Autodesk Fusion 360 part; units mm, degrees
(part 3 of 6)
sketch "Sketch27" plane through (0, 0, 4) normal (0, 0, 1) x (1, 0, 0)
  arc A0 (9.3874, -0.8005) -> (9.3971, -0.6778) centre (0, 0) ccw
  spline S0 degree 3 poles (9.5677, -0.4943) (9.542, -0.4981) (9.5172, -0.5068) (9.4723, -0.5334) (9.4527, -0.5509) (9.4254, -0.587) (9.4161, -0.6039) (9.4026, -0.6398) (9.3985, -0.6587) (9.3971, -0.6778) knots 0 0 0 0 0.007813 0.007813 0.015626 0.015626 0.021388 0.021388 0.027151 0.027151 0.027151 0.027151
  spline S1 degree 5 poles (9.5677, -0.4943) (9.5692, -0.4941) (9.5738, -0.4934) (9.5816, -0.4923) (9.5926, -0.4906) (9.6069, -0.4883) (9.6229, -0.4856) (9.6389, -0.4827) (9.6549, -0.4797) (9.6709, -0.4766) (9.6869, -0.4734) (9.7029, -0.4701) (9.7189, -0.4667) (9.7349, -0.4631) (9.7509, -0.4595) (9.7669, -0.4557) (9.7829, -0.4519) (9.7989, -0.4479) (9.8149, -0.4439) (9.8309, -0.4397) (9.8469, -0.4355) (9.8629, -0.4311) (9.8788, -0.4267) (9.8948, -0.4222) (9.9108, -0.4176) (9.9268, -0.4129) (9.9428, -0.4081) (9.9587, -0.4032) (9.9747, -0.3982) (9.9906, -0.3931) (10.0066, -0.388) (10.0225, -0.3828) (10.0385, -0.3775) (10.0544, -0.3721) (10.0704, -0.3666) (10.0863, -0.3611) (10.1022, -0.3554) (10.1181, -0.3497) (10.1341, -0.3439) (10.15, -0.338) (10.1659, -0.3321) (10.1818, -0.3261) (10.1977, -0.32) (10.2136, -0.3138) (10.2294, -0.3075) (10.2453, -0.3012) (10.2612, -0.2948) (10.277, -0.2883) (10.2929, -0.2818) (10.3087, -0.2752) (10.3246, -0.2685) (10.3404, -0.2617) (10.3562, -0.2549) (10.372, -0.248) (10.3878, -0.241) (10.4036, -0.2339) (10.4194, -0.2268) (10.4352, -0.2196) (10.451, -0.2124) (10.4668, -0.205) (10.4794, -0.1991) (10.4888, -0.1946) (10.4951, -0.1917) (10.4983, -0.1902) knots 0.165068 0.165068 0.165068 0.165068 0.165068 0.165068 0.171429 0.185714 0.2 0.214286 0.228571 0.242857 0.257143 0.271429 0.285714 0.3 0.314286 0.328571 0.342857 0.357143 0.371429 0.385714 0.4 0.414286 0.428571 0.442857 0.457143 0.471429 0.485714 0.5 0.514286 0.528571 0.542857 0.557143 0.571429 0.585714 0.6 0.614286 0.628571 0.642857 0.657143 0.671429 0.685714 0.7 0.714286 0.728571 0.742857 0.757143 0.771429 0.785714 0.8 0.814286 0.828571 0.842857 0.857143 0.871429 0.885714 0.9 0.914286 0.928571 0.942857 0.957143 0.971429 0.985714 1 1 1 1 1 1
  arc A1 (10.4983, -0.1902) -> (10.4983, 0.1902) centre (0, 0) ccw
  spline S2 degree 5 poles (10.4983, 0.1902) (10.4951, 0.1917) (10.4888, 0.1946) (10.4794, 0.1991) (10.4668, 0.205) (10.451, 0.2124) (10.4352, 0.2196) (10.4194, 0.2268) (10.4036, 0.2339) (10.3878, 0.241) (10.372, 0.248) (10.3562, 0.2549) (10.3404, 0.2617) (10.3246, 0.2685) (10.3087, 0.2752) (10.2929, 0.2818) (10.277, 0.2883) (10.2612, 0.2948) (10.2453, 0.3012) (10.2294, 0.3075) (10.2136, 0.3138) (10.1977, 0.32) (10.1818, 0.3261) (10.1659, 0.3321) (10.15, 0.338) (10.1341, 0.3439) (10.1181, 0.3497) (10.1022, 0.3554) (10.0863, 0.3611) (10.0704, 0.3666) (10.0544, 0.3721) (10.0385, 0.3775) (10.0225, 0.3828) (10.0066, 0.388) (9.9906, 0.3931) (9.9747, 0.3982) (9.9587, 0.4032) (9.9428, 0.4081) (9.9268, 0.4129) (9.9108, 0.4176) (9.8948, 0.4222) (9.8788, 0.4267) (9.8629, 0.4311) (9.8469, 0.4355) (9.8309, 0.4397) (9.8149, 0.4439) (9.7989, 0.4479) (9.7829, 0.4519) (9.7669, 0.4557) (9.7509, 0.4595) (9.7349, 0.4631) (9.7189, 0.4667) (9.7029, 0.4701) (9.6869, 0.4734) (9.6709, 0.4766) (9.6549, 0.4797) (9.6389, 0.4827) (9.6229, 0.4856) (9.6069, 0.4883) (9.5926, 0.4906) (9.5816, 0.4923) (9.5738, 0.4934) (9.5692, 0.4941) (9.5677, 0.4943) knots -1 -1 -1 -1 -1 -1 -0.985714 -0.971429 -0.957143 -0.942857 -0.928571 -0.914286 -0.9 -0.885714 -0.871429 -0.857143 -0.842857 -0.828571 -0.814286 -0.8 -0.785714 -0.771429 -0.757143 -0.742857 -0.728571 -0.714286 -0.7 -0.685714 -0.671429 -0.657143 -0.642857 -0.628571 -0.614286 -0.6 -0.585714 -0.571429 -0.557143 -0.542857 -0.528571 -0.514286 -0.5 -0.485714 -0.471429 -0.457143 -0.442857 -0.428571 -0.414286 -0.4 -0.385714 -0.371429 -0.357143 -0.342857 -0.328571 -0.314286 -0.3 -0.285714 -0.271429 -0.257143 -0.242857 -0.228571 -0.214286 -0.2 -0.185714 -0.171429 -0.165068 -0.165068 -0.165068 -0.165068 -0.165068 -0.165068
  spline S3 degree 3 poles (9.3971, 0.6778) (9.399, 0.6519) (9.4059, 0.6265) (9.4291, 0.5799) (9.4451, 0.559) (9.4791, 0.5292) (9.4953, 0.5187) (9.5302, 0.5026) (9.5487, 0.4971) (9.5677, 0.4943) knots 0 0 0 0 0.007813 0.007813 0.015626 0.015626 0.021388 0.021388 0.027151 0.027151 0.027151 0.027151
  arc A2 (9.3971, 0.6778) -> (9.3874, 0.8005) centre (0, 0) ccw
  spline S4 degree 3 poles (9.5273, 1.0085) (9.5024, 1.0007) (9.4793, 0.9882) (9.4391, 0.955) (9.4225, 0.9347) (9.4012, 0.8947) (9.3947, 0.8766) (9.3869, 0.8389) (9.3858, 0.8197) (9.3874, 0.8005) knots 0 0 0 0 0.007813 0.007813 0.015626 0.015626 0.021388 0.021388 0.027151 0.027151 0.027151 0.027151
  spline S5 degree 5 poles (9.5273, 1.0085) (9.5286, 1.0089) (9.5331, 1.0103) (9.5406, 1.0127) (9.5513, 1.0161) (9.565, 1.0206) (9.5803, 1.0258) (9.5957, 1.0311) (9.6111, 1.0365) (9.6264, 1.0421) (9.6417, 1.0478) (9.657, 1.0535) (9.6722, 1.0594) (9.6875, 1.0654) (9.7027, 1.0715) (9.7179, 1.0777) (9.7331, 1.0841) (9.7483, 1.0905) (9.7635, 1.097) (9.7786, 1.1036) (9.7938, 1.1103) (9.8089, 1.1171) (9.824, 1.1239) (9.839, 1.1309) (9.8541, 1.138) (9.8691, 1.1451) (9.8842, 1.1524) (9.8992, 1.1597) (9.9142, 1.1671) (9.9291, 1.1746) (9.9441, 1.1821) (9.959, 1.1898) (9.9739, 1.1975) (9.9889, 1.2054) (10.0037, 1.2133) (10.0186, 1.2212) (10.0335, 1.2293) (10.0483, 1.2374) (10.0631, 1.2456) (10.0779, 1.2539) (10.0927, 1.2623) (10.1074, 1.2707) (10.1222, 1.2792) (10.1369, 1.2878) (10.1516, 1.2965) (10.1663, 1.3052) (10.181, 1.314) (10.1956, 1.3229) (10.2102, 1.3318) (10.2249, 1.3409) (10.2395, 1.35) (10.254, 1.3591) (10.2686, 1.3683) (10.2831, 1.3776) (10.2977, 1.387) (10.3122, 1.3964) (10.3266, 1.4059) (10.3411, 1.4155) (10.3556, 1.4252) (10.37, 1.4349) (10.3815, 1.4427) (10.3901, 1.4486) (10.3959, 1.4525) (10.3988, 1.4545) knots 0.165068 0.165068 0.165068 0.165068 0.165068 0.165068 0.171429 0.185714 0.2 0.214286 0.228571 0.242857 0.257143 0.271429 0.285714 0.3 0.314286 0.328571 0.342857 0.357143 0.371429 0.385714 0.4 0.414286 0.428571 0.442857 0.457143 0.471429 0.485714 0.5 0.514286 0.528571 0.542857 0.557143 0.571429 0.585714 0.6 0.614286 0.628571 0.642857 0.657143 0.671429 0.685714 0.7 0.714286 0.728571 0.742857 0.757143 0.771429 0.785714 0.8 0.814286 0.828571 0.842857 0.857143 0.871429 0.885714 0.9 0.914286 0.928571 0.942857 0.957143 0.971429 0.985714 1 1 1 1 1 1
  arc A3 (10.3988, 1.4545) -> (10.3393, 1.8301) centre (0, 0) ccw
  spline S6 degree 5 poles (10.3393, 1.8301) (10.3359, 1.8311) (10.3292, 1.8331) (10.3192, 1.836) (10.3058, 1.8399) (10.2891, 1.8446) (10.2724, 1.8493) (10.2557, 1.854) (10.239, 1.8585) (10.2223, 1.863) (10.2056, 1.8674) (10.1888, 1.8718) (10.1722, 1.8761) (10.1555, 1.8803) (10.1388, 1.8844) (10.1221, 1.8885) (10.1054, 1.8925) (10.0887, 1.8964) (10.072, 1.9002) (10.0554, 1.904) (10.0387, 1.9077) (10.0221, 1.9113) (10.0054, 1.9148) (9.9888, 1.9183) (9.9721, 1.9217) (9.9555, 1.925) (9.9389, 1.9282) (9.9223, 1.9314) (9.9056, 1.9345) (9.889, 1.9374) (9.8724, 1.9404) (9.8559, 1.9432) (9.8393, 1.9459) (9.8227, 1.9486) (9.8061, 1.9512) (9.7896, 1.9537) (9.773, 1.9561) (9.7565, 1.9584) (9.74, 1.9607) (9.7235, 1.9628) (9.707, 1.9649) (9.6905, 1.9668) (9.674, 1.9687) (9.6575, 1.9705) (9.6411, 1.9722) (9.6246, 1.9738) (9.6082, 1.9753) (9.5918, 1.9767) (9.5754, 1.978) (9.559, 1.9792) (9.5426, 1.9803) (9.5262, 1.9813) (9.5099, 1.9822) (9.4936, 1.983) (9.4773, 1.9836) (9.461, 1.9842) (9.4447, 1.9846) (9.4284, 1.9849) (9.4122, 1.9851) (9.3978, 1.9851) (9.3866, 1.9851) (9.3787, 1.985) (9.374, 1.985) (9.3726, 1.985) knots -1 -1 -1 -1 -1 -1 -0.985714 -0.971429 -0.957143 -0.942857 -0.928571 -0.914286 -0.9 -0.885714 -0.871429 -0.857143 -0.842857 -0.828571 -0.814286 -0.8 -0.785714 -0.771429 -0.757143 -0.742857 -0.728571 -0.714286 -0.7 -0.685714 -0.671429 -0.657143 -0.642857 -0.628571 -0.614286 -0.6 -0.585714 -0.571429 -0.557143 -0.542857 -0.528571 -0.514286 -0.5 -0.485714 -0.471429 -0.457143 -0.442857 -0.428571 -0.414286 -0.4 -0.385714 -0.371429 -0.357143 -0.342857 -0.328571 -0.314286 -0.3 -0.285714 -0.271429 -0.257143 -0.242857 -0.228571 -0.214286 -0.2 -0.185714 -0.171429 -0.165068 -0.165068 -0.165068 -0.165068 -0.165068 -0.165068
  spline S7 degree 3 poles (9.1754, 2.1395) (9.1813, 2.1142) (9.1921, 2.0902) (9.2223, 2.0478) (9.2414, 2.0297) (9.2796, 2.0056) (9.2973, 1.9977) (9.3343, 1.9873) (9.3534, 1.9847) (9.3726, 1.985) knots 0 0 0 0 0.007813 0.007813 0.015626 0.015626 0.021388 0.021388 0.027151 0.027151 0.027151 0.027151
  arc A4 (9.1754, 2.1395) -> (9.1466, 2.2592) centre (0, 0) ccw
  spline S8 degree 3 poles (9.2522, 2.4865) (9.2289, 2.4749) (9.208, 2.4589) (9.1735, 2.4199) (9.1603, 2.3971) (9.1455, 2.3544) (9.1419, 2.3354) (9.1401, 2.297) (9.142, 2.2778) (9.1466, 2.2592) knots 0 0 0 0 0.007813 0.007813 0.015626 0.015626 0.021388 0.021388 0.027151 0.027151 0.027151 0.027151
  spline S9 degree 5 poles (9.2522, 2.4865) (9.2535, 2.4871) (9.2577, 2.4892) (9.2648, 2.4927) (9.2747, 2.4977) (9.2875, 2.5043) (9.3019, 2.5118) (9.3163, 2.5195) (9.3306, 2.5273) (9.3448, 2.5351) (9.3591, 2.5431) (9.3733, 2.5513) (9.3874, 2.5595) (9.4016, 2.5678) (9.4156, 2.5762) (9.4297, 2.5847) (9.4437, 2.5933) (9.4577, 2.602) (9.4717, 2.6108) (9.4856, 2.6197) (9.4995, 2.6287) (9.5134, 2.6378) (9.5272, 2.6469) (9.541, 2.6562) (9.5548, 2.6655) (9.5685, 2.6749) (9.5822, 2.6844) (9.5959, 2.694) (9.6095, 2.7036) (9.6232, 2.7134) (9.6367, 2.7232) (9.6503, 2.7331) (9.6638, 2.7431) (9.6773, 2.7531) (9.6908, 2.7632) (9.7042, 2.7735) (9.7176, 2.7837) (9.731, 2.7941) (9.7443, 2.8045) (9.7577, 2.815) (9.7709, 2.8256) (9.7842, 2.8362) (9.7974, 2.8469) (9.8106, 2.8577) (9.8238, 2.8686) (9.8369, 2.8795) (9.8501, 2.8905) (9.8631, 2.9016) (9.8762, 2.9127) (9.8892, 2.9239) (9.9022, 2.9351) (9.9152, 2.9465) (9.9281, 2.9579) (9.941, 2.9693) (9.9539, 2.9808) (9.9667, 2.9924) (9.9796, 3.0041) (9.9924, 3.0158) (10.0051, 3.0276) (10.0178, 3.0394) (10.028, 3.0489) (10.0356, 3.0561) (10.0407, 3.0609) (10.0432, 3.0633) knots 0.165068 0.165068 0.165068 0.165068 0.165068 0.165068 0.171429 0.185714 0.2 0.214286 0.228571 0.242857 0.257143 0.271429 0.285714 0.3 0.314286 0.328571 0.342857 0.357143 0.371429 0.385714 0.4 0.414286 0.428571 0.442857 0.457143 0.471429 0.485714 0.5 0.514286 0.528571 0.542857 0.557143 0.571429 0.585714 0.6 0.614286 0.628571 0.642857 0.657143 0.671429 0.685714 0.7 0.714286 0.728571 0.742857 0.757143 0.771429 0.785714 0.8 0.814286 0.828571 0.842857 0.857143 0.871429 0.885714 0.9 0.914286 0.928571 0.942857 0.957143 0.971429 0.985714 1 1 1 1 1 1
  arc A5 (10.0432, 3.0633) -> (9.9257, 3.425) centre (0, 0) ccw
  spline S10 degree 5 poles (9.9257, 3.425) (9.9222, 3.4254) (9.9153, 3.4263) (9.9049, 3.4277) (9.8911, 3.4294) (9.8739, 3.4315) (9.8566, 3.4335) (9.8394, 3.4355) (9.8222, 3.4374) (9.805, 3.4392) (9.7878, 3.441) (9.7706, 3.4426) (9.7534, 3.4443) (9.7363, 3.4458) (9.7192, 3.4473) (9.702, 3.4487) (9.6849, 3.45) (9.6679, 3.4513) (9.6508, 3.4524) (9.6337, 3.4536) (9.6167, 3.4546) (9.5997, 3.4556) (9.5827, 3.4565) (9.5657, 3.4573) (9.5487, 3.458) (9.5318, 3.4587) (9.5149, 3.4593) (9.498, 3.4598) (9.4811, 3.4602) (9.4642, 3.4606) (9.4474, 3.4609) (9.4305, 3.4611) (9.4137, 3.4612) (9.3969, 3.4612) (9.3802, 3.4612) (9.3634, 3.4611) (9.3467, 3.4609) (9.33, 3.4606) (9.3133, 3.4602) (9.2967, 3.4597) (9.2801, 3.4592) (9.2635, 3.4586) (9.2469, 3.4578) (9.2304, 3.457) (9.2138, 3.4561) (9.1973, 3.4551) (9.1809, 3.454) (9.1644, 3.4529) (9.148, 3.4516) (9.1317, 3.4502) (9.1153, 3.4487) (9.099, 3.4471) (9.0827, 3.4455) (9.0665, 3.4437) (9.0503, 3.4418) (9.0341, 3.4398) (9.0179, 3.4377) (9.0018, 3.4354) (8.9858, 3.4331) (8.9715, 3.4308) (8.9605, 3.4291) (8.9527, 3.4278) (8.9481, 3.427) (8.9467, 3.4267) knots -1 -1 -1 -1 -1 -1 -0.985714 -0.971429 -0.957143 -0.942857 -0.928571 -0.914286 -0.9 -0.885714 -0.871429 -0.857143 -0.842857 -0.828571 -0.814286 -0.8 -0.785714 -0.771429 -0.757143 -0.742857 -0.728571 -0.714286 -0.7 -0.685714 -0.671429 -0.657143 -0.642857 -0.628571 -0.614286 -0.6 -0.585714 -0.571429 -0.557143 -0.542857 -0.528571 -0.514286 -0.5 -0.485714 -0.471429 -0.457143 -0.442857 -0.428571 -0.414286 -0.4 -0.385714 -0.371429 -0.357143 -0.342857 -0.328571 -0.314286 -0.3 -0.285714 -0.271429 -0.257143 -0.242857 -0.228571 -0.214286 -0.2 -0.185714 -0.171429 -0.165068 -0.165068 -0.165068 -0.165068 -0.165068 -0.165068
  spline S11 degree 3 poles (8.7277, 3.5485) (8.7375, 3.5244) (8.7519, 3.5024) (8.7884, 3.4652) (8.8101, 3.4504) (8.8517, 3.4325) (8.8703, 3.4275) (8.9085, 3.423) (8.9278, 3.4235) (8.9467, 3.4267) knots 0 0 0 0 0.007813 0.007813 0.015626 0.015626 0.021388 0.021388 0.027151 0.027151 0.027151 0.027151
  arc A6 (8.7277, 3.5485) -> (8.6806, 3.6622) centre (0, 0) ccw
  spline S12 degree 3 poles (8.7493, 3.9032) (8.7281, 3.8882) (8.71, 3.8691) (8.682, 3.8251) (8.6725, 3.8006) (8.6646, 3.7561) (8.664, 3.7368) (8.6683, 3.6986) (8.6731, 3.6799) (8.6806, 3.6622) knots 0 0 0 0 0.007813 0.007813 0.015626 0.015626 0.021388 0.021388 0.027151 0.027151 0.027151 0.027151
  spline S13 degree 5 poles (8.7493, 3.9032) (8.7505, 3.904) (8.7543, 3.9067) (8.7608, 3.9113) (8.7698, 3.9179) (8.7814, 3.9264) (8.7945, 3.9361) (8.8074, 3.9459) (8.8204, 3.9558) (8.8332, 3.9658) (8.846, 3.9759) (8.8588, 3.9861) (8.8715, 3.9965) (8.8841, 4.0069) (8.8967, 4.0174) (8.9093, 4.028) (8.9218, 4.0387) (8.9342, 4.0495) (8.9467, 4.0604) (8.959, 4.0713) (8.9713, 4.0824) (8.9836, 4.0935) (8.9958, 4.1047) (9.008, 4.116) (9.0202, 4.1274) (9.0323, 4.1388) (9.0443, 4.1503) (9.0563, 4.1619) (9.0683, 4.1736) (9.0802, 4.1854) (9.0921, 4.1972) (9.1039, 4.2091) (9.1157, 4.221) (9.1275, 4.2331) (9.1392, 4.2452) (9.1509, 4.2574) (9.1625, 4.2696) (9.1741, 4.282) (9.1856, 4.2943) (9.1972, 4.3068) (9.2086, 4.3193) (9.2201, 4.3319) (9.2314, 4.3445) (9.2428, 4.3573) (9.2541, 4.37) (9.2654, 4.3829) (9.2766, 4.3958) (9.2878, 4.4088) (9.299, 4.4218) (9.3101, 4.4349) (9.3211, 4.448) (9.3322, 4.4613) (9.3432, 4.4745) (9.3541, 4.4879) (9.365, 4.5013) (9.3759, 4.5147) (9.3868, 4.5282) (9.3976, 4.5418) (9.4083, 4.5554) (9.419, 4.5691) (9.4276, 4.5801) (9.434, 4.5884) (9.4382, 4.5939) (9.4404, 4.5967) knots 0.165068 0.165068 0.165068 0.165068 0.165068 0.165068 0.171429 0.185714 0.2 0.214286 0.228571 0.242857 0.257143 0.271429 0.285714 0.3 0.314286 0.328571 0.342857 0.357143 0.371429 0.385714 0.4 0.414286 0.428571 0.442857 0.457143 0.471429 0.485714 0.5 0.514286 0.528571 0.542857 0.557143 0.571429 0.585714 0.6 0.614286 0.628571 0.642857 0.657143 0.671429 0.685714 0.7 0.714286 0.728571 0.742857 0.757143 0.771429 0.785714 0.8 0.814286 0.828571 0.842857 0.857143 0.871429 0.885714 0.9 0.914286 0.928571 0.942857 0.957143 0.971429 0.985714 1 1 1 1 1 1
  arc A7 (9.4404, 4.5967) -> (9.2677, 4.9355) centre (0, 0) ccw
  spline S14 degree 5 poles (9.2677, 4.9355) (9.2642, 4.9355) (9.2572, 4.9353) (9.2468, 4.935) (9.2329, 4.9345) (9.2155, 4.9339) (9.1981, 4.9332) (9.1808, 4.9324) (9.1635, 4.9316) (9.1462, 4.9307) (9.129, 4.9297) (9.1118, 4.9287) (9.0946, 4.9276) (9.0774, 4.9265) (9.0602, 4.9252) (9.0431, 4.9239) (9.026, 4.9226) (9.0089, 4.9212) (8.9919, 4.9197) (8.9749, 4.9181) (8.9579, 4.9164) (8.9409, 4.9147) (8.924, 4.913) (8.9071, 4.9111) (8.8902, 4.9092) (8.8734, 4.9072) (8.8566, 4.9051) (8.8398, 4.903) (8.823, 4.9008) (8.8063, 4.8985) (8.7896, 4.8961) (8.773, 4.8937) (8.7564, 4.8912) (8.7398, 4.8886) (8.7232, 4.886) (8.7067, 4.8832) (8.6902, 4.8804) (8.6738, 4.8775) (8.6574, 4.8745) (8.641, 4.8715) (8.6247, 4.8683) (8.6084, 4.8651) (8.5921, 4.8618) (8.5759, 4.8584) (8.5597, 4.8549) (8.5436, 4.8514) (8.5275, 4.8477) (8.5115, 4.844) (8.4955, 4.8401) (8.4795, 4.8362) (8.4636, 4.8322) (8.4477, 4.8281) (8.4319, 4.8239) (8.4161, 4.8196) (8.4004, 4.8152) (8.3848, 4.8107) (8.3691, 4.8061) (8.3536, 4.8013) (8.3381, 4.7965) (8.3244, 4.7921) (8.3138, 4.7886) (8.3063, 4.7861) (8.3018, 4.7846) (8.3005, 4.7841) knots -1 -1 -1 -1 -1 -1 -0.985714 -0.971429 -0.957143 -0.942857 -0.928571 -0.914286 -0.9 -0.885714 -0.871429 -0.857143 -0.842857 -0.828571 -0.814286 -0.8 -0.785714 -0.771429 -0.757143 -0.742857 -0.728571 -0.714286 -0.7 -0.685714 -0.671429 -0.657143 -0.642857 -0.628571 -0.614286 -0.6 -0.585714 -0.571429 -0.557143 -0.542857 -0.528571 -0.514286 -0.5 -0.485714 -0.471429 -0.457143 -0.442857 -0.428571 -0.414286 -0.4 -0.385714 -0.371429 -0.357143 -0.342857 -0.328571 -0.314286 -0.3 -0.285714 -0.271429 -0.257143 -0.242857 -0.228571 -0.214286 -0.2 -0.185714 -0.171429 -0.165068 -0.165068 -0.165068 -0.165068 -0.165068 -0.165068
  spline S15 degree 3 poles (8.0651, 4.8702) (8.0786, 4.8479) (8.0963, 4.8284) (8.1381, 4.7974) (8.1619, 4.7861) (8.2057, 4.775) (8.2249, 4.7729) (8.2633, 4.7744) (8.2823, 4.7779) (8.3005, 4.7841) knots 0 0 0 0 0.007813 0.007813 0.015626 0.015626 0.021388 0.021388 0.027151 0.027151 0.027151 0.027151
  arc A8 (8.0651, 4.8702) -> (8.0008, 4.9751) centre (0, 0) ccw
  spline S16 degree 3 poles (8.031, 5.2238) (8.0124, 5.2057) (7.9975, 5.184) (7.9768, 5.1362) (7.9712, 5.1105) (7.9703, 5.0653) (7.9727, 5.0461) (7.9829, 5.0091) (7.9907, 4.9914) (8.0008, 4.9751) knots 0 0 0 0 0.007813 0.007813 0.015626 0.015626 0.021388 0.021388 0.027151 0.027151 0.027151 0.027151
  spline S17 degree 5 poles (8.031, 5.2238) (8.032, 5.2249) (8.0354, 5.2281) (8.041, 5.2337) (8.0489, 5.2415) (8.0591, 5.2517) (8.0705, 5.2634) (8.0817, 5.2751) (8.0929, 5.2869) (8.1041, 5.2988) (8.1151, 5.3108) (8.1261, 5.3229) (8.1371, 5.3351) (8.1479, 5.3473) (8.1587, 5.3597) (8.1695, 5.3721) (8.1801, 5.3847) (8.1908, 5.3973) (8.2013, 5.4099) (8.2118, 5.4227) (8.2223, 5.4355) (8.2326, 5.4484) (8.243, 5.4614) (8.2532, 5.4745) (8.2634, 5.4876) (8.2736, 5.5008) (8.2837, 5.5141) (8.2938, 5.5274) (8.3037, 5.5408) (8.3137, 5.5543) (8.3236, 5.5678) (8.3334, 5.5814) (8.3432, 5.5951) (8.3529, 5.6088) (8.3626, 5.6226) (8.3722, 5.6365) (8.3818, 5.6504) (8.3913, 5.6644) (8.4008, 5.6784) (8.4102, 5.6925) (8.4196, 5.7067) (8.4289, 5.7209) (8.4382, 5.7352) (8.4474, 5.7495) (8.4565, 5.7639) (8.4657, 5.7784) (8.4747, 5.7929) (8.4838, 5.8074) (8.4927, 5.822) (8.5017, 5.8367) (8.5106, 5.8514) (8.5194, 5.8662) (8.5282, 5.881) (8.5369, 5.8959) (8.5456, 5.9109) (8.5542, 5.9259) (8.5628, 5.9409) (8.5714, 5.956) (8.5799, 5.9711) (8.5883, 5.9863) (8.595, 5.9985) (8.6001, 6.0077) (8.6034, 6.0138) (8.6051, 6.0169) knots 0.165068 0.165068 0.165068 0.165068 0.165068 0.165068 0.171429 0.185714 0.2 0.214286 0.228571 0.242857 0.257143 0.271429 0.285714 0.3 0.314286 0.328571 0.342857 0.357143 0.371429 0.385714 0.4 0.414286 0.428571 0.442857 0.457143 0.471429 0.485714 0.5 0.514286 0.528571 0.542857 0.557143 0.571429 0.585714 0.6 0.614286 0.628571 0.642857 0.657143 0.671429 0.685714 0.7 0.714286 0.728571 0.742857 0.757143 0.771429 0.785714 0.8 0.814286 0.828571 0.842857 0.857143 0.871429 0.885714 0.9 0.914286 0.928571 0.942857 0.957143 0.971429 0.985714 1 1 1 1 1 1
  arc A9 (8.6051, 6.0169) -> (8.3815, 6.3246) centre (0, 0) ccw
  spline S18 degree 5 poles (8.3815, 6.3246) (8.3781, 6.3239) (8.3712, 6.3227) (8.361, 6.3207) (8.3473, 6.3181) (8.3302, 6.3147) (8.3132, 6.3113) (8.2962, 6.3079) (8.2792, 6.3044) (8.2623, 6.3008) (8.2454, 6.2971) (8.2286, 6.2934) (8.2117, 6.2897) (8.1949, 6.2858) (8.1782, 6.2819) (8.1615, 6.278) (8.1448, 6.274) (8.1282, 6.2699) (8.1116, 6.2657) (8.095, 6.2615) (8.0785, 6.2572) (8.062, 6.2529) (8.0456, 6.2485) (8.0292, 6.244) (8.0128, 6.2395) (7.9965, 6.2349) (7.9802, 6.2302) (7.964, 6.2255) (7.9478, 6.2207) (7.9316, 6.2158) (7.9155, 6.2109) (7.8994, 6.2059) (7.8834, 6.2008) (7.8674, 6.1956) (7.8515, 6.1904) (7.8356, 6.1851) (7.8198, 6.1798) (7.804, 6.1743) (7.7883, 6.1688) (7.7726, 6.1632) (7.7569, 6.1576) (7.7413, 6.1519) (7.7258, 6.146) (7.7103, 6.1402) (7.6949, 6.1342) (7.6795, 6.1282) (7.6642, 6.122) (7.6489, 6.1158) (7.6337, 6.1095) (7.6186, 6.1032) (7.6035, 6.0967) (7.5884, 6.0902) (7.5735, 6.0835) (7.5586, 6.0768) (7.5437, 6.07) (7.529, 6.0631) (7.5143, 6.0561) (7.4997, 6.049) (7.4851, 6.0418) (7.4723, 6.0353) (7.4623, 6.0302) (7.4553, 6.0265) (7.4512, 6.0244) (7.4499, 6.0237) knots -1 -1 -1 -1 -1 -1 -0.985714 -0.971429 -0.957143 -0.942857 -0.928571 -0.914286 -0.9 -0.885714 -0.871429 -0.857143 -0.842857 -0.828571 -0.814286 -0.8 -0.785714 -0.771429 -0.757143 -0.742857 -0.728571 -0.714286 -0.7 -0.685714 -0.671429 -0.657143 -0.642857 -0.628571 -0.614286 -0.6 -0.585714 -0.571429 -0.557143 -0.542857 -0.528571 -0.514286 -0.5 -0.485714 -0.471429 -0.457143 -0.442857 -0.428571 -0.414286 -0.4 -0.385714 -0.371429 -0.357143 -0.342857 -0.328571 -0.314286 -0.3 -0.285714 -0.271429 -0.257143 -0.242857 -0.228571 -0.214286 -0.2 -0.185714 -0.171429 -0.165068 -0.165068 -0.165068 -0.165068 -0.165068 -0.165068
  spline S19 degree 3 poles (7.204, 6.0719) (7.2208, 6.0519) (7.2413, 6.0355) (7.2874, 6.0114) (7.3127, 6.004) (7.3577, 5.9998) (7.377, 6.0008) (7.4147, 6.0083) (7.4329, 6.0148) (7.4499, 6.0237) knots 0 0 0 0 0.007813 0.007813 0.015626 0.015626 0.021388 0.021388 0.027151 0.027151 0.027151 0.027151
  arc A10 (7.204, 6.0719) -> (7.1241, 6.1654) centre (0, 0) ccw
  spline S20 degree 3 poles (7.1149, 6.4159) (7.0994, 6.395) (7.088, 6.3713) (7.0751, 6.3208) (7.0736, 6.2946) (7.0798, 6.2497) (7.0852, 6.2312) (7.1011, 6.1962) (7.1115, 6.18) (7.1241, 6.1654) knots 0 0 0 0 0.007813 0.007813 0.015626 0.015626 0.021388 0.021388 0.027151 0.027151 0.027151 0.027151
  spline S21 degree 5 poles (7.1149, 6.4159) (7.1158, 6.417) (7.1186, 6.4208) (7.1233, 6.4271) (7.1299, 6.4361) (7.1383, 6.4478) (7.1477, 6.4611) (7.157, 6.4744) (7.1663, 6.4878) (7.1754, 6.5013) (7.1844, 6.5149) (7.1934, 6.5286) (7.2023, 6.5423) (7.2111, 6.5561) (7.2198, 6.57) (7.2285, 6.584) (7.2371, 6.598) (7.2456, 6.6121) (7.254, 6.6263) (7.2624, 6.6405) (7.2707, 6.6549) (7.279, 6.6692) (7.2871, 6.6837) (7.2952, 6.6982) (7.3033, 6.7127) (7.3112, 6.7274) (7.3191, 6.742) (7.327, 6.7568) (7.3347, 6.7716) (7.3424, 6.7865) (7.3501, 6.8014) (7.3577, 6.8163) (7.3652, 6.8314) (7.3727, 6.8465) (7.3801, 6.8616) (7.3874, 6.8768) (7.3947, 6.892) (7.4019, 6.9073) (7.409, 6.9227) (7.4161, 6.9381) (7.4232, 6.9535) (7.4302, 6.969) (7.4371, 6.9846) (7.444, 7.0002) (7.4508, 7.0158) (7.4575, 7.0315) (7.4642, 7.0473) (7.4708, 7.0631) (7.4774, 7.0789) (7.4839, 7.0948) (7.4904, 7.1107) (7.4968, 7.1267) (7.5032, 7.1427) (7.5095, 7.1588) (7.5157, 7.1749) (7.5219, 7.1911) (7.528, 7.2073) (7.5341, 7.2235) (7.5401, 7.2398) (7.5461, 7.2561) (7.5508, 7.2692) (7.5544, 7.2791) (7.5567, 7.2857) (7.5579, 7.2889) knots 0.165068 0.165068 0.165068 0.165068 0.165068 0.165068 0.171429 0.185714 0.2 0.214286 0.228571 0.242857 0.257143 0.271429 0.285714 0.3 0.314286 0.328571 0.342857 0.357143 0.371429 0.385714 0.4 0.414286 0.428571 0.442857 0.457143 0.471429 0.485714 0.5 0.514286 0.528571 0.542857 0.557143 0.571429 0.585714 0.6 0.614286 0.628571 0.642857 0.657143 0.671429 0.685714 0.7 0.714286 0.728571 0.742857 0.757143 0.771429 0.785714 0.8 0.814286 0.828571 0.842857 0.857143 0.871429 0.885714 0.9 0.914286 0.928571 0.942857 0.957143 0.971429 0.985714 1 1 1 1 1 1
  arc A11 (7.5579, 7.2889) -> (7.2889, 7.5579) centre (0, 0) ccw
  spline S22 degree 5 poles (7.2889, 7.5579) (7.2857, 7.5567) (7.2791, 7.5544) (7.2692, 7.5508) (7.2561, 7.5461) (7.2398, 7.5401) (7.2235, 7.5341) (7.2073, 7.528) (7.1911, 7.5219) (7.1749, 7.5157) (7.1588, 7.5095) (7.1427, 7.5032) (7.1267, 7.4968) (7.1107, 7.4904) (7.0948, 7.4839) (7.0789, 7.4774) (7.0631, 7.4708) (7.0473, 7.4642) (7.0315, 7.4575) (7.0158, 7.4508) (7.0002, 7.444) (6.9846, 7.4371) (6.969, 7.4302) (6.9535, 7.4232) (6.9381, 7.4161) (6.9227, 7.409) (6.9073, 7.4019) (6.892, 7.3947) (6.8768, 7.3874) (6.8616, 7.3801) (6.8465, 7.3727) (6.8314, 7.3652) (6.8163, 7.3577) (6.8014, 7.3501) (6.7865, 7.3424) (6.7716, 7.3347) (6.7568, 7.327) (6.742, 7.3191) (6.7274, 7.3112) (6.7127, 7.3033) (6.6982, 7.2952) (6.6837, 7.2871) (6.6692, 7.279) (6.6549, 7.2707) (6.6405, 7.2624) (6.6263, 7.254) (6.6121, 7.2456) (6.598, 7.2371) (6.584, 7.2285) (6.57, 7.2198) (6.5561, 7.2111) (6.5423, 7.2023) (6.5286, 7.1934) (6.5149, 7.1844) (6.5013, 7.1754) (6.4878, 7.1663) (6.4744, 7.157) (6.4611, 7.1477) (6.4478, 7.1383) (6.4361, 7.1299) (6.4271, 7.1233) (6.4208, 7.1186) (6.417, 7.1158) (6.4159, 7.1149) knots -1 -1 -1 -1 -1 -1 -0.985714 -0.971429 -0.957143 -0.942857 -0.928571 -0.914286 -0.9 -0.885714 -0.871429 -0.857143 -0.842857 -0.828571 -0.814286 -0.8 -0.785714 -0.771429 -0.757143 -0.742857 -0.728571 -0.714286 -0.7 -0.685714 -0.671429 -0.657143 -0.642857 -0.628571 -0.614286 -0.6 -0.585714 -0.571429 -0.557143 -0.542857 -0.528571 -0.514286 -0.5 -0.485714 -0.471429 -0.457143 -0.442857 -0.428571 -0.414286 -0.4 -0.385714 -0.371429 -0.357143 -0.342857 -0.328571 -0.314286 -0.3 -0.285714 -0.271429 -0.257143 -0.242857 -0.228571 -0.214286 -0.2 -0.185714 -0.171429 -0.165068 -0.165068 -0.165068 -0.165068 -0.165068 -0.165068
  spline S23 degree 3 poles (6.1654, 7.1241) (6.1851, 7.107) (6.208, 7.094) (6.2573, 7.0774) (6.2834, 7.074) (6.3286, 7.077) (6.3474, 7.081) (6.3835, 7.0943) (6.4005, 7.1035) (6.4159, 7.1149) knots 0 0 0 0 0.007813 0.007813 0.015626 0.015626 0.021388 0.021388 0.027151 0.027151 0.027151 0.027151
  arc A12 (6.1654, 7.1241) -> (6.0719, 7.204) centre (0, 0) ccw
  spline S24 degree 3 poles (6.0237, 7.4499) (6.0116, 7.4268) (6.0041, 7.4016) (5.9992, 7.3498) (6.0018, 7.3236) (6.015, 7.2803) (6.0232, 7.2629) (6.0443, 7.2308) (6.0572, 7.2163) (6.0719, 7.204) knots 0 0 0 0 0.007813 0.007813 0.015626 0.015626 0.021388 0.021388 0.027151 0.027151 0.027151 0.027151
  spline S25 degree 5 poles (6.0237, 7.4499) (6.0244, 7.4512) (6.0265, 7.4553) (6.0302, 7.4623) (6.0353, 7.4723) (6.0418, 7.4851) (6.049, 7.4997) (6.0561, 7.5143) (6.0631, 7.529) (6.07, 7.5437) (6.0768, 7.5586) (6.0835, 7.5735) (6.0902, 7.5884) (6.0967, 7.6035) (6.1032, 7.6186) (6.1095, 7.6337) (6.1158, 7.6489) (6.122, 7.6642) (6.1282, 7.6795) (6.1342, 7.6949) (6.1402, 7.7103) (6.146, 7.7258) (6.1519, 7.7413) (6.1576, 7.7569) (6.1632, 7.7726) (6.1688, 7.7883) (6.1743, 7.804) (6.1798, 7.8198) (6.1851, 7.8356) (6.1904, 7.8515) (6.1956, 7.8674) (6.2008, 7.8834) (6.2059, 7.8994) (6.2109, 7.9155) (6.2158, 7.9316) (6.2207, 7.9478) (6.2255, 7.964) (6.2302, 7.9802) (6.2349, 7.9965) (6.2395, 8.0128) (6.244, 8.0292) (6.2485, 8.0456) (6.2529, 8.062) (6.2572, 8.0785) (6.2615, 8.095) (6.2657, 8.1116) (6.2699, 8.1282) (6.274, 8.1448) (6.278, 8.1615) (6.2819, 8.1782) (6.2858, 8.1949) (6.2897, 8.2117) (6.2934, 8.2286) (6.2971, 8.2454) (6.3008, 8.2623) (6.3044, 8.2792) (6.3079, 8.2962) (6.3113, 8.3132) (6.3147, 8.3302) (6.3181, 8.3473) (6.3207, 8.361) (6.3227, 8.3712) (6.3239, 8.3781) (6.3246, 8.3815) knots 0.165068 0.165068 0.165068 0.165068 0.165068 0.165068 0.171429 0.185714 0.2 0.214286 0.228571 0.242857 0.257143 0.271429 0.285714 0.3 0.314286 0.328571 0.342857 0.357143 0.371429 0.385714 0.4 0.414286 0.428571 0.442857 0.457143 0.471429 0.485714 0.5 0.514286 0.528571 0.542857 0.557143 0.571429 0.585714 0.6 0.614286 0.628571 0.642857 0.657143 0.671429 0.685714 0.7 0.714286 0.728571 0.742857 0.757143 0.771429 0.785714 0.8 0.814286 0.828571 0.842857 0.857143 0.871429 0.885714 0.9 0.914286 0.928571 0.942857 0.957143 0.971429 0.985714 1 1 1 1 1 1
  arc A13 (6.3246, 8.3815) -> (6.0169, 8.6051) centre (0, 0) ccw
  spline S26 degree 5 poles (6.0169, 8.6051) (6.0138, 8.6034) (6.0077, 8.6001) (5.9985, 8.595) (5.9863, 8.5883) (5.9711, 8.5799) (5.956, 8.5714) (5.9409, 8.5628) (5.9259, 8.5542) (5.9109, 8.5456) (5.8959, 8.5369) (5.881, 8.5282) (5.8662, 8.5194) (5.8514, 8.5106) (5.8367, 8.5017) (5.822, 8.4927) (5.8074, 8.4838) (5.7929, 8.4747) (5.7784, 8.4657) (5.7639, 8.4565) (5.7495, 8.4474) (5.7352, 8.4382) (5.7209, 8.4289) (5.7067, 8.4196) (5.6925, 8.4102) (5.6784, 8.4008) (5.6644, 8.3913) (5.6504, 8.3818) (5.6365, 8.3722) (5.6226, 8.3626) (5.6088, 8.3529) (5.5951, 8.3432) (5.5814, 8.3334) (5.5678, 8.3236) (5.5543, 8.3137) (5.5408, 8.3037) (5.5274, 8.2938) (5.5141, 8.2837) (5.5008, 8.2736) (5.4876, 8.2634) (5.4745, 8.2532) (5.4614, 8.243) (5.4484, 8.2326) (5.4355, 8.2223) (5.4227, 8.2118) (5.4099, 8.2013) (5.3973, 8.1908) (5.3847, 8.1801) (5.3721, 8.1695) (5.3597, 8.1587) (5.3473, 8.1479) (5.3351, 8.1371) (5.3229, 8.1261) (5.3108, 8.1151) (5.2988, 8.1041) (5.2869, 8.0929) (5.2751, 8.0817) (5.2634, 8.0705) (5.2517, 8.0591) (5.2415, 8.0489) (5.2337, 8.041) (5.2281, 8.0354) (5.2249, 8.032) (5.2238, 8.031) knots -1 -1 -1 -1 -1 -1 -0.985714 -0.971429 -0.957143 -0.942857 -0.928571 -0.914286 -0.9 -0.885714 -0.871429 -0.857143 -0.842857 -0.828571 -0.814286 -0.8 -0.785714 -0.771429 -0.757143 -0.742857 -0.728571 -0.714286 -0.7 -0.685714 -0.671429 -0.657143 -0.642857 -0.628571 -0.614286 -0.6 -0.585714 -0.571429 -0.557143 -0.542857 -0.528571 -0.514286 -0.5 -0.485714 -0.471429 -0.457143 -0.442857 -0.428571 -0.414286 -0.4 -0.385714 -0.371429 -0.357143 -0.342857 -0.328571 -0.314286 -0.3 -0.285714 -0.271429 -0.257143 -0.242857 -0.228571 -0.214286 -0.2 -0.185714 -0.171429 -0.165068 -0.165068 -0.165068 -0.165068 -0.165068 -0.165068
  spline S27 degree 3 poles (4.9751, 8.0008) (4.9972, 7.9871) (5.0218, 7.9778) (5.0731, 7.9691) (5.0994, 7.9699) (5.1436, 7.9798) (5.1616, 7.9868) (5.1951, 8.0055) (5.2104, 8.0173) (5.2238, 8.031) knots 0 0 0 0 0.007813 0.007813 0.015626 0.015626 0.021388 0.021388 0.027151 0.027151 0.027151 0.027151
  arc A14 (4.9751, 8.0008) -> (4.8702, 8.0651) centre (0, 0) ccw
  spline S28 degree 3 poles (4.7841, 8.3005) (4.7758, 8.2758) (4.7723, 8.2498) (4.7756, 8.1978) (4.7823, 8.1724) (4.802, 8.1316) (4.8129, 8.1157) (4.8388, 8.0873) (4.8537, 8.0751) (4.8702, 8.0651) knots 0 0 0 0 0.007813 0.007813 0.015626 0.015626 0.021388 0.021388 0.027151 0.027151 0.027151 0.027151
  spline S29 degree 5 poles (4.7841, 8.3005) (4.7846, 8.3018) (4.7861, 8.3063) (4.7886, 8.3138) (4.7921, 8.3244) (4.7965, 8.3381) (4.8013, 8.3536) (4.8061, 8.3691) (4.8107, 8.3848) (4.8152, 8.4004) (4.8196, 8.4161) (4.8239, 8.4319) (4.8281, 8.4477) (4.8322, 8.4636) (4.8362, 8.4795) (4.8401, 8.4955) (4.844, 8.5115) (4.8477, 8.5275) (4.8514, 8.5436) (4.8549, 8.5597) (4.8584, 8.5759) (4.8618, 8.5921) (4.8651, 8.6084) (4.8683, 8.6247) (4.8715, 8.641) (4.8745, 8.6574) (4.8775, 8.6738) (4.8804, 8.6902) (4.8832, 8.7067) (4.886, 8.7232) (4.8886, 8.7398) (4.8912, 8.7564) (4.8937, 8.773) (4.8961, 8.7896) (4.8985, 8.8063) (4.9008, 8.823) (4.903, 8.8398) (4.9051, 8.8566) (4.9072, 8.8734) (4.9092, 8.8902) (4.9111, 8.9071) (4.913, 8.924) (4.9147, 8.9409) (4.9164, 8.9579) (4.9181, 8.9749) (4.9197, 8.9919) (4.9212, 9.0089) (4.9226, 9.026) (4.9239, 9.0431) (4.9252, 9.0602) (4.9265, 9.0774) (4.9276, 9.0946) (4.9287, 9.1118) (4.9297, 9.129) (4.9307, 9.1462) (4.9316, 9.1635) (4.9324, 9.1808) (4.9332, 9.1981) (4.9339, 9.2155) (4.9345, 9.2329) (4.935, 9.2468) (4.9353, 9.2572) (4.9355, 9.2642) (4.9355, 9.2677) knots 0.165068 0.165068 0.165068 0.165068 0.165068 0.165068 0.171429 0.185714 0.2 0.214286 0.228571 0.242857 0.257143 0.271429 0.285714 0.3 0.314286 0.328571 0.342857 0.357143 0.371429 0.385714 0.4 0.414286 0.428571 0.442857 0.457143 0.471429 0.485714 0.5 0.514286 0.528571 0.542857 0.557143 0.571429 0.585714 0.6 0.614286 0.628571 0.642857 0.657143 0.671429 0.685714 0.7 0.714286 0.728571 0.742857 0.757143 0.771429 0.785714 0.8 0.814286 0.828571 0.842857 0.857143 0.871429 0.885714 0.9 0.914286 0.928571 0.942857 0.957143 0.971429 0.985714 1 1 1 1 1 1
  arc A15 (4.9355, 9.2677) -> (4.5967, 9.4404) centre (0, 0) ccw
  spline S30 degree 5 poles (4.5967, 9.4404) (4.5939, 9.4382) (4.5884, 9.434) (4.5801, 9.4276) (4.5691, 9.419) (4.5554, 9.4083) (4.5418, 9.3976) (4.5282, 9.3868) (4.5147, 9.3759) (4.5013, 9.365) (4.4879, 9.3541) (4.4745, 9.3432) (4.4613, 9.3322) (4.448, 9.3211) (4.4349, 9.3101) (4.4218, 9.299) (4.4088, 9.2878) (4.3958, 9.2766) (4.3829, 9.2654) (4.37, 9.2541) (4.3573, 9.2428) (4.3445, 9.2314) (4.3319, 9.2201) (4.3193, 9.2086) (4.3068, 9.1972) (4.2943, 9.1856) (4.282, 9.1741) (4.2696, 9.1625) (4.2574, 9.1509) (4.2452, 9.1392) (4.2331, 9.1275) (4.221, 9.1157) (4.2091, 9.1039) (4.1972, 9.0921) (4.1854, 9.0802) (4.1736, 9.0683) (4.1619, 9.0563) (4.1503, 9.0443) (4.1388, 9.0323) (4.1274, 9.0202) (4.116, 9.008) (4.1047, 8.9958) (4.0935, 8.9836) (4.0824, 8.9713) (4.0713, 8.959) (4.0604, 8.9467) (4.0495, 8.9342) (4.0387, 8.9218) (4.028, 8.9093) (4.0174, 8.8967) (4.0069, 8.8841) (3.9965, 8.8715) (3.9861, 8.8588) (3.9759, 8.846) (3.9658, 8.8332) (3.9558, 8.8204) (3.9459, 8.8074) (3.9361, 8.7945) (3.9264, 8.7814) (3.9179, 8.7698) (3.9113, 8.7608) (3.9067, 8.7543) (3.904, 8.7505) (3.9032, 8.7493) knots -1 -1 -1 -1 -1 -1 -0.985714 -0.971429 -0.957143 -0.942857 -0.928571 -0.914286 -0.9 -0.885714 -0.871429 -0.857143 -0.842857 -0.828571 -0.814286 -0.8 -0.785714 -0.771429 -0.757143 -0.742857 -0.728571 -0.714286 -0.7 -0.685714 -0.671429 -0.657143 -0.642857 -0.628571 -0.614286 -0.6 -0.585714 -0.571429 -0.557143 -0.542857 -0.528571 -0.514286 -0.5 -0.485714 -0.471429 -0.457143 -0.442857 -0.428571 -0.414286 -0.4 -0.385714 -0.371429 -0.357143 -0.342857 -0.328571 -0.314286 -0.3 -0.285714 -0.271429 -0.257143 -0.242857 -0.228571 -0.214286 -0.2 -0.185714 -0.171429 -0.165068 -0.165068 -0.165068 -0.165068 -0.165068 -0.165068
  spline S31 degree 3 poles (3.6622, 8.6806) (3.6862, 8.6705) (3.712, 8.6651) (3.764, 8.6646) (3.7899, 8.6695) (3.8319, 8.6862) (3.8486, 8.6959) (3.8788, 8.7197) (3.8921, 8.7336) (3.9032, 8.7493) knots 0 0 0 0 0.007813 0.007813 0.015626 0.015626 0.021388 0.021388 0.027151 0.027151 0.027151 0.027151
  arc A16 (3.6622, 8.6806) -> (3.5485, 8.7277) centre (0, 0) ccw
  spline S32 degree 3 poles (3.4267, 8.9467) (3.4223, 8.921) (3.423, 8.8947) (3.4344, 8.8439) (3.445, 8.8198) (3.4709, 8.7827) (3.4841, 8.7687) (3.5141, 8.7447) (3.5307, 8.7349) (3.5485, 8.7277) knots 0 0 0 0 0.007813 0.007813 0.015626 0.015626 0.021388 0.021388 0.027151 0.027151 0.027151 0.027151
  spline S33 degree 5 poles (3.4267, 8.9467) (3.427, 8.9481) (3.4278, 8.9527) (3.4291, 8.9605) (3.4308, 8.9715) (3.4331, 8.9858) (3.4354, 9.0018) (3.4377, 9.0179) (3.4398, 9.0341) (3.4418, 9.0503) (3.4437, 9.0665) (3.4455, 9.0827) (3.4471, 9.099) (3.4487, 9.1153) (3.4502, 9.1317) (3.4516, 9.148) (3.4529, 9.1644) (3.454, 9.1809) (3.4551, 9.1973) (3.4561, 9.2138) (3.457, 9.2304) (3.4578, 9.2469) (3.4586, 9.2635) (3.4592, 9.2801) (3.4597, 9.2967) (3.4602, 9.3133) (3.4606, 9.33) (3.4609, 9.3467) (3.4611, 9.3634) (3.4612, 9.3802) (3.4612, 9.3969) (3.4612, 9.4137) (3.4611, 9.4305) (3.4609, 9.4474) (3.4606, 9.4642) (3.4602, 9.4811) (3.4598, 9.498) (3.4593, 9.5149) (3.4587, 9.5318) (3.458, 9.5487) (3.4573, 9.5657) (3.4565, 9.5827) (3.4556, 9.5997) (3.4546, 9.6167) (3.4536, 9.6337) (3.4524, 9.6508) (3.4513, 9.6679) (3.45, 9.6849) (3.4487, 9.702) (3.4473, 9.7192) (3.4458, 9.7363) (3.4443, 9.7534) (3.4426, 9.7706) (3.441, 9.7878) (3.4392, 9.805) (3.4374, 9.8222) (3.4355, 9.8394) (3.4335, 9.8566) (3.4315, 9.8739) (3.4294, 9.8911) (3.4277, 9.9049) (3.4263, 9.9153) (3.4254, 9.9222) (3.425, 9.9257) knots 0.165068 0.165068 0.165068 0.165068 0.165068 0.165068 0.171429 0.185714 0.2 0.214286 0.228571 0.242857 0.257143 0.271429 0.285714 0.3 0.314286 0.328571 0.342857 0.357143 0.371429 0.385714 0.4 0.414286 0.428571 0.442857 0.457143 0.471429 0.485714 0.5 0.514286 0.528571 0.542857 0.557143 0.571429 0.585714 0.6 0.614286 0.628571 0.642857 0.657143 0.671429 0.685714 0.7 0.714286 0.728571 0.742857 0.757143 0.771429 0.785714 0.8 0.814286 0.828571 0.842857 0.857143 0.871429 0.885714 0.9 0.914286 0.928571 0.942857 0.957143 0.971429 0.985714 1 1 1 1 1 1
  arc A17 (3.425, 9.9257) -> (3.0633, 10.0432) centre (0, 0) ccw
  spline S34 degree 5 poles (3.0633, 10.0432) (3.0609, 10.0407) (3.0561, 10.0356) (3.0489, 10.028) (3.0394, 10.0178) (3.0276, 10.0051) (3.0158, 9.9924) (3.0041, 9.9796) (2.9924, 9.9667) (2.9808, 9.9539) (2.9693, 9.941) (2.9579, 9.9281) (2.9465, 9.9152) (2.9351, 9.9022) (2.9239, 9.8892) (2.9127, 9.8762) (2.9016, 9.8631) (2.8905, 9.8501) (2.8795, 9.8369) (2.8686, 9.8238) (2.8577, 9.8106) (2.8469, 9.7974) (2.8362, 9.7842) (2.8256, 9.7709) (2.815, 9.7577) (2.8045, 9.7443) (2.7941, 9.731) (2.7837, 9.7176) (2.7735, 9.7042) (2.7632, 9.6908) (2.7531, 9.6773) (2.7431, 9.6638) (2.7331, 9.6503) (2.7232, 9.6367) (2.7134, 9.6232) (2.7036, 9.6095) (2.694, 9.5959) (2.6844, 9.5822) (2.6749, 9.5685) (2.6655, 9.5548) (2.6562, 9.541) (2.6469, 9.5272) (2.6378, 9.5134) (2.6287, 9.4995) (2.6197, 9.4856) (2.6108, 9.4717) (2.602, 9.4577) (2.5933, 9.4437) (2.5847, 9.4297) (2.5762, 9.4156) (2.5678, 9.4016) (2.5595, 9.3874) (2.5513, 9.3733) (2.5431, 9.3591) (2.5351, 9.3448) (2.5273, 9.3306) (2.5195, 9.3163) (2.5118, 9.3019) (2.5043, 9.2875) (2.4977, 9.2747) (2.4927, 9.2648) (2.4892, 9.2577) (2.4871, 9.2535) (2.4865, 9.2522) knots -1 -1 -1 -1 -1 -1 -0.985714 -0.971429 -0.957143 -0.942857 -0.928571 -0.914286 -0.9 -0.885714 -0.871429 -0.857143 -0.842857 -0.828571 -0.814286 -0.8 -0.785714 -0.771429 -0.757143 -0.742857 -0.728571 -0.714286 -0.7 -0.685714 -0.671429 -0.657143 -0.642857 -0.628571 -0.614286 -0.6 -0.585714 -0.571429 -0.557143 -0.542857 -0.528571 -0.514286 -0.5 -0.485714 -0.471429 -0.457143 -0.442857 -0.428571 -0.414286 -0.4 -0.385714 -0.371429 -0.357143 -0.342857 -0.328571 -0.314286 -0.3 -0.285714 -0.271429 -0.257143 -0.242857 -0.228571 -0.214286 -0.2 -0.185714 -0.171429 -0.165068 -0.165068 -0.165068 -0.165068 -0.165068 -0.165068
  spline S35 degree 3 poles (2.2592, 9.1466) (2.2845, 9.1404) (2.3107, 9.1391) (2.3623, 9.1468) (2.387, 9.1556) (2.4259, 9.1787) (2.4409, 9.1909) (2.467, 9.2191) (2.4779, 9.235) (2.4865, 9.2522) knots 0 0 0 0 0.007813 0.007813 0.015626 0.015626 0.021388 0.021388 0.027151 0.027151 0.027151 0.027151
  arc A18 (2.2592, 9.1466) -> (2.1395, 9.1754) centre (0, 0) ccw
  spline S36 degree 3 poles (1.985, 9.3726) (1.9846, 9.3466) (1.9894, 9.3207) (2.0086, 9.2723) (2.0228, 9.2502) (2.0542, 9.2176) (2.0694, 9.2057) (2.1028, 9.1867) (2.1208, 9.1797) (2.1395, 9.1754) knots 0 0 0 0 0.007813 0.007813 0.015626 0.015626 0.021388 0.021388 0.027151 0.027151 0.027151 0.027151
  spline S37 degree 5 poles (1.985, 9.3726) (1.985, 9.374) (1.985, 9.3787) (1.9851, 9.3866) (1.9851, 9.3978) (1.9851, 9.4122) (1.9849, 9.4284) (1.9846, 9.4447) (1.9842, 9.461) (1.9836, 9.4773) (1.983, 9.4936) (1.9822, 9.5099) (1.9813, 9.5262) (1.9803, 9.5426) (1.9792, 9.559) (1.978, 9.5754) (1.9767, 9.5918) (1.9753, 9.6082) (1.9738, 9.6246) (1.9722, 9.6411) (1.9705, 9.6575) (1.9687, 9.674) (1.9668, 9.6905) (1.9649, 9.707) (1.9628, 9.7235) (1.9607, 9.74) (1.9584, 9.7565) (1.9561, 9.773) (1.9537, 9.7896) (1.9512, 9.8061) (1.9486, 9.8227) (1.9459, 9.8393) (1.9432, 9.8559) (1.9404, 9.8724) (1.9374, 9.889) (1.9345, 9.9056) (1.9314, 9.9223) (1.9282, 9.9389) (1.925, 9.9555) (1.9217, 9.9721) (1.9183, 9.9888) (1.9148, 10.0054) (1.9113, 10.0221) (1.9077, 10.0387) (1.904, 10.0554) (1.9002, 10.072) (1.8964, 10.0887) (1.8925, 10.1054) (1.8885, 10.1221) (1.8844, 10.1388) (1.8803, 10.1555) (1.8761, 10.1722) (1.8718, 10.1888) (1.8674, 10.2056) (1.863, 10.2223) (1.8585, 10.239) (1.854, 10.2557) (1.8493, 10.2724) (1.8446, 10.2891) (1.8399, 10.3058) (1.836, 10.3192) (1.8331, 10.3292) (1.8311, 10.3359) (1.8301, 10.3393) knots 0.165068 0.165068 0.165068 0.165068 0.165068 0.165068 0.171429 0.185714 0.2 0.214286 0.228571 0.242857 0.257143 0.271429 0.285714 0.3 0.314286 0.328571 0.342857 0.357143 0.371429 0.385714 0.4 0.414286 0.428571 0.442857 0.457143 0.471429 0.485714 0.5 0.514286 0.528571 0.542857 0.557143 0.571429 0.585714 0.6 0.614286 0.628571 0.642857 0.657143 0.671429 0.685714 0.7 0.714286 0.728571 0.742857 0.757143 0.771429 0.785714 0.8 0.814286 0.828571 0.842857 0.857143 0.871429 0.885714 0.9 0.914286 0.928571 0.942857 0.957143 0.971429 0.985714 1 1 1 1 1 1
  arc A19 (1.8301, 10.3393) -> (1.4545, 10.3988) centre (0, 0) ccw
  spline S38 degree 5 poles (1.4545, 10.3988) (1.4525, 10.3959) (1.4486, 10.3901) (1.4427, 10.3815) (1.4349, 10.37) (1.4252, 10.3556) (1.4155, 10.3411) (1.4059, 10.3266) (1.3964, 10.3122) (1.387, 10.2977) (1.3776, 10.2831) (1.3683, 10.2686) (1.3591, 10.254) (1.35, 10.2395) (1.3409, 10.2249) (1.3318, 10.2102) (1.3229, 10.1956) (1.314, 10.181) (1.3052, 10.1663) (1.2965, 10.1516) (1.2878, 10.1369) (1.2792, 10.1222) (1.2707, 10.1074) (1.2623, 10.0927) (1.2539, 10.0779) (1.2456, 10.0631) (1.2374, 10.0483) (1.2293, 10.0335) (1.2212, 10.0186) (1.2133, 10.0037) (1.2054, 9.9889) (1.1975, 9.9739) (1.1898, 9.959) (1.1821, 9.9441) (1.1746, 9.9291) (1.1671, 9.9142) (1.1597, 9.8992) (1.1524, 9.8842) (1.1451, 9.8691) (1.138, 9.8541) (1.1309, 9.839) (1.1239, 9.824) (1.1171, 9.8089) (1.1103, 9.7938) (1.1036, 9.7786) (1.097, 9.7635) (1.0905, 9.7483) (1.0841, 9.7331) (1.0777, 9.7179) (1.0715, 9.7027) (1.0654, 9.6875) (1.0594, 9.6722) (1.0535, 9.657) (1.0478, 9.6417) (1.0421, 9.6264) (1.0365, 9.6111) (1.0311, 9.5957) (1.0258, 9.5803) (1.0206, 9.565) (1.0161, 9.5513) (1.0127, 9.5406) (1.0103, 9.5331) (1.0089, 9.5286) (1.0085, 9.5273) knots -1 -1 -1 -1 -1 -1 -0.985714 -0.971429 -0.957143 -0.942857 -0.928571 -0.914286 -0.9 -0.885714 -0.871429 -0.857143 -0.842857 -0.828571 -0.814286 -0.8 -0.785714 -0.771429 -0.757143 -0.742857 -0.728571 -0.714286 -0.7 -0.685714 -0.671429 -0.657143 -0.642857 -0.628571 -0.614286 -0.6 -0.585714 -0.571429 -0.557143 -0.542857 -0.528571 -0.514286 -0.5 -0.485714 -0.471429 -0.457143 -0.442857 -0.428571 -0.414286 -0.4 -0.385714 -0.371429 -0.357143 -0.342857 -0.328571 -0.314286 -0.3 -0.285714 -0.271429 -0.257143 -0.242857 -0.228571 -0.214286 -0.2 -0.185714 -0.171429 -0.165068 -0.165068 -0.165068 -0.165068 -0.165068 -0.165068
  spline S39 degree 3 poles (0.8005, 9.3874) (0.8265, 9.3852) (0.8526, 9.3881) (0.9023, 9.4037) (0.9254, 9.4163) (0.9602, 9.4452) (0.9731, 9.4596) (0.9944, 9.4915) (1.0028, 9.5089) (1.0085, 9.5273) knots 0 0 0 0 0.007813 0.007813 0.015626 0.015626 0.021388 0.021388 0.027151 0.027151 0.027151 0.027151
  arc A20 (0.8005, 9.3874) -> (0.6778, 9.3971) centre (0, 0) ccw
  spline S40 degree 3 poles (0.4943, 9.5677) (0.4981, 9.542) (0.5068, 9.5172) (0.5334, 9.4723) (0.5509, 9.4527) (0.587, 9.4254) (0.6039, 9.4161) (0.6398, 9.4026) (0.6587, 9.3985) (0.6778, 9.3971) knots 0 0 0 0 0.007813 0.007813 0.015626 0.015626 0.021388 0.021388 0.027151 0.027151 0.027151 0.027151
  spline S41 degree 5 poles (0.4943, 9.5677) (0.4941, 9.5692) (0.4934, 9.5738) (0.4923, 9.5816) (0.4906, 9.5926) (0.4883, 9.6069) (0.4856, 9.6229) (0.4827, 9.6389) (0.4797, 9.6549) (0.4766, 9.6709) (0.4734, 9.6869) (0.4701, 9.7029) (0.4667, 9.7189) (0.4631, 9.7349) (0.4595, 9.7509) (0.4557, 9.7669) (0.4519, 9.7829) (0.4479, 9.7989) (0.4439, 9.8149) (0.4397, 9.8309) (0.4355, 9.8469) (0.4311, 9.8629) (0.4267, 9.8788) (0.4222, 9.8948) (0.4176, 9.9108) (0.4129, 9.9268) (0.4081, 9.9428) (0.4032, 9.9587) (0.3982, 9.9747) (0.3931, 9.9906) (0.388, 10.0066) (0.3828, 10.0225) (0.3775, 10.0385) (0.3721, 10.0544) (0.3666, 10.0704) (0.3611, 10.0863) (0.3554, 10.1022) (0.3497, 10.1181) (0.3439, 10.1341) (0.338, 10.15) (0.3321, 10.1659) (0.3261, 10.1818) (0.32, 10.1977) (0.3138, 10.2136) (0.3075, 10.2294) (0.3012, 10.2453) (0.2948, 10.2612) (0.2883, 10.277) (0.2818, 10.2929) (0.2752, 10.3087) (0.2685, 10.3246) (0.2617, 10.3404) (0.2549, 10.3562) (0.248, 10.372) (0.241, 10.3878) (0.2339, 10.4036) (0.2268, 10.4194) (0.2196, 10.4352) (0.2124, 10.451) (0.205, 10.4668) (0.1991, 10.4794) (0.1946, 10.4888) (0.1917, 10.4951) (0.1902, 10.4983) knots 0.165068 0.165068 0.165068 0.165068 0.165068 0.165068 0.171429 0.185714 0.2 0.214286 0.228571 0.242857 0.257143 0.271429 0.285714 0.3 0.314286 0.328571 0.342857 0.357143 0.371429 0.385714 0.4 0.414286 0.428571 0.442857 0.457143 0.471429 0.485714 0.5 0.514286 0.528571 0.542857 0.557143 0.571429 0.585714 0.6 0.614286 0.628571 0.642857 0.657143 0.671429 0.685714 0.7 0.714286 0.728571 0.742857 0.757143 0.771429 0.785714 0.8 0.814286 0.828571 0.842857 0.857143 0.871429 0.885714 0.9 0.914286 0.928571 0.942857 0.957143 0.971429 0.985714 1 1 1 1 1 1
  arc A21 (0.1902, 10.4983) -> (-0.1902, 10.4983) centre (0, 0) ccw
  spline S42 degree 5 poles (-0.1902, 10.4983) (-0.1917, 10.4951) (-0.1946, 10.4888) (-0.1991, 10.4794) (-0.205, 10.4668) (-0.2124, 10.451) (-0.2196, 10.4352) (-0.2268, 10.4194) (-0.2339, 10.4036) (-0.241, 10.3878) (-0.248, 10.372) (-0.2549, 10.3562) (-0.2617, 10.3404) (-0.2685, 10.3246) (-0.2752, 10.3087) (-0.2818, 10.2929) (-0.2883, 10.277) (-0.2948, 10.2612) (-0.3012, 10.2453) (-0.3075, 10.2294) (-0.3138, 10.2136) (-0.32, 10.1977) (-0.3261, 10.1818) (-0.3321, 10.1659) (-0.338, 10.15) (-0.3439, 10.1341) (-0.3497, 10.1181) (-0.3554, 10.1022) (-0.3611, 10.0863) (-0.3666, 10.0704) (-0.3721, 10.0544) (-0.3775, 10.0385) (-0.3828, 10.0225) (-0.388, 10.0066) (-0.3931, 9.9906) (-0.3982, 9.9747) (-0.4032, 9.9587) (-0.4081, 9.9428) (-0.4129, 9.9268) (-0.4176, 9.9108) (-0.4222, 9.8948) (-0.4267, 9.8788) (-0.4311, 9.8629) (-0.4355, 9.8469) (-0.4397, 9.8309) (-0.4439, 9.8149) (-0.4479, 9.7989) (-0.4519, 9.7829) (-0.4557, 9.7669) (-0.4595, 9.7509) (-0.4631, 9.7349) (-0.4667, 9.7189) (-0.4701, 9.7029) (-0.4734, 9.6869) (-0.4766, 9.6709) (-0.4797, 9.6549) (-0.4827, 9.6389) (-0.4856, 9.6229) (-0.4883, 9.6069) (-0.4906, 9.5926) (-0.4923, 9.5816) (-0.4934, 9.5738) (-0.4941, 9.5692) (-0.4943, 9.5677) knots -1 -1 -1 -1 -1 -1 -0.985714 -0.971429 -0.957143 -0.942857 -0.928571 -0.914286 -0.9 -0.885714 -0.871429 -0.857143 -0.842857 -0.828571 -0.814286 -0.8 -0.785714 -0.771429 -0.757143 -0.742857 -0.728571 -0.714286 -0.7 -0.685714 -0.671429 -0.657143 -0.642857 -0.628571 -0.614286 -0.6 -0.585714 -0.571429 -0.557143 -0.542857 -0.528571 -0.514286 -0.5 -0.485714 -0.471429 -0.457143 -0.442857 -0.428571 -0.414286 -0.4 -0.385714 -0.371429 -0.357143 -0.342857 -0.328571 -0.314286 -0.3 -0.285714 -0.271429 -0.257143 -0.242857 -0.228571 -0.214286 -0.2 -0.185714 -0.171429 -0.165068 -0.165068 -0.165068 -0.165068 -0.165068 -0.165068
  spline S43 degree 3 poles (-0.6778, 9.3971) (-0.6519, 9.399) (-0.6265, 9.4059) (-0.5799, 9.4291) (-0.559, 9.4451) (-0.5292, 9.4791) (-0.5187, 9.4953) (-0.5026, 9.5302) (-0.4971, 9.5487) (-0.4943, 9.5677) knots 0 0 0 0 0.007813 0.007813 0.015626 0.015626 0.021388 0.021388 0.027151 0.027151 0.027151 0.027151
  arc A22 (-0.6778, 9.3971) -> (-0.8005, 9.3874) centre (0, 0) ccw
  spline S44 degree 3 poles (-1.0085, 9.5273) (-1.0007, 9.5024) (-0.9882, 9.4793) (-0.955, 9.4391) (-0.9347, 9.4225) (-0.8947, 9.4012) (-0.8766, 9.3947) (-0.8389, 9.3869) (-0.8197, 9.3858) (-0.8005, 9.3874) knots 0 0 0 0 0.007813 0.007813 0.015626 0.015626 0.021388 0.021388 0.027151 0.027151 0.027151 0.027151
  spline S45 degree 5 poles (-1.0085, 9.5273) (-1.0089, 9.5286) (-1.0103, 9.5331) (-1.0127, 9.5406) (-1.0161, 9.5513) (-1.0206, 9.565) (-1.0258, 9.5803) (-1.0311, 9.5957) (-1.0365, 9.6111) (-1.0421, 9.6264) (-1.0478, 9.6417) (-1.0535, 9.657) (-1.0594, 9.6722) (-1.0654, 9.6875) (-1.0715, 9.7027) (-1.0777, 9.7179) (-1.0841, 9.7331) (-1.0905, 9.7483) (-1.097, 9.7635) (-1.1036, 9.7786) (-1.1103, 9.7938) (-1.1171, 9.8089) (-1.1239, 9.824) (-1.1309, 9.839) (-1.138, 9.8541) (-1.1451, 9.8691) (-1.1524, 9.8842) (-1.1597, 9.8992) (-1.1671, 9.9142) (-1.1746, 9.9291) (-1.1821, 9.9441) (-1.1898, 9.959) (-1.1975, 9.9739) (-1.2054, 9.9889) (-1.2133, 10.0037) (-1.2212, 10.0186) (-1.2293, 10.0335) (-1.2374, 10.0483) (-1.2456, 10.0631) (-1.2539, 10.0779) (-1.2623, 10.0927) (-1.2707, 10.1074) (-1.2792, 10.1222) (-1.2878, 10.1369) (-1.2965, 10.1516) (-1.3052, 10.1663) (-1.314, 10.181) (-1.3229, 10.1956) (-1.3318, 10.2102) (-1.3409, 10.2249) (-1.35, 10.2395) (-1.3591, 10.254) (-1.3683, 10.2686) (-1.3776, 10.2831) (-1.387, 10.2977) (-1.3964, 10.3122) (-1.4059, 10.3266) (-1.4155, 10.3411) (-1.4252, 10.3556) (-1.4349, 10.37) (-1.4427, 10.3815) (-1.4486, 10.3901) (-1.4525, 10.3959) (-1.4545, 10.3988) knots 0.165068 0.165068 0.165068 0.165068 0.165068 0.165068 0.171429 0.185714 0.2 0.214286 0.228571 0.242857 0.257143 0.271429 0.285714 0.3 0.314286 0.328571 0.342857 0.357143 0.371429 0.385714 0.4 0.414286 0.428571 0.442857 0.457143 0.471429 0.485714 0.5 0.514286 0.528571 0.542857 0.557143 0.571429 0.585714 0.6 0.614286 0.628571 0.642857 0.657143 0.671429 0.685714 0.7 0.714286 0.728571 0.742857 0.757143 0.771429 0.785714 0.8 0.814286 0.828571 0.842857 0.857143 0.871429 0.885714 0.9 0.914286 0.928571 0.942857 0.957143 0.971429 0.985714 1 1 1 1 1 1
  arc A23 (-1.4545, 10.3988) -> (-1.8301, 10.3393) centre (0, 0) ccw
  spline S46 degree 5 poles (-1.8301, 10.3393) (-1.8311, 10.3359) (-1.8331, 10.3292) (-1.836, 10.3192) (-1.8399, 10.3058) (-1.8446, 10.2891) (-1.8493, 10.2724) (-1.854, 10.2557) (-1.8585, 10.239) (-1.863, 10.2223) (-1.8674, 10.2056) (-1.8718, 10.1888) (-1.8761, 10.1722) (-1.8803, 10.1555) (-1.8844, 10.1388) (-1.8885, 10.1221) (-1.8925, 10.1054) (-1.8964, 10.0887) (-1.9002, 10.072) (-1.904, 10.0554) (-1.9077, 10.0387) (-1.9113, 10.0221) (-1.9148, 10.0054) (-1.9183, 9.9888) (-1.9217, 9.9721) (-1.925, 9.9555) (-1.9282, 9.9389) (-1.9314, 9.9223) (-1.9345, 9.9056) (-1.9374, 9.889) (-1.9404, 9.8724) (-1.9432, 9.8559) (-1.9459, 9.8393) (-1.9486, 9.8227) (-1.9512, 9.8061) (-1.9537, 9.7896) (-1.9561, 9.773) (-1.9584, 9.7565) (-1.9607, 9.74) (-1.9628, 9.7235) (-1.9649, 9.707) (-1.9668, 9.6905) (-1.9687, 9.674) (-1.9705, 9.6575) (-1.9722, 9.6411) (-1.9738, 9.6246) (-1.9753, 9.6082) (-1.9767, 9.5918) (-1.978, 9.5754) (-1.9792, 9.559) (-1.9803, 9.5426) (-1.9813, 9.5262) (-1.9822, 9.5099) (-1.983, 9.4936) (-1.9836, 9.4773) (-1.9842, 9.461) (-1.9846, 9.4447) (-1.9849, 9.4284) (-1.9851, 9.4122) (-1.9851, 9.3978) (-1.9851, 9.3866) (-1.985, 9.3787) (-1.985, 9.374) (-1.985, 9.3726) knots -1 -1 -1 -1 -1 -1 -0.985714 -0.971429 -0.957143 -0.942857 -0.928571 -0.914286 -0.9 -0.885714 -0.871429 -0.857143 -0.842857 -0.828571 -0.814286 -0.8 -0.785714 -0.771429 -0.757143 -0.742857 -0.728571 -0.714286 -0.7 -0.685714 -0.671429 -0.657143 -0.642857 -0.628571 -0.614286 -0.6 -0.585714 -0.571429 -0.557143 -0.542857 -0.528571 -0.514286 -0.5 -0.485714 -0.471429 -0.457143 -0.442857 -0.428571 -0.414286 -0.4 -0.385714 -0.371429 -0.357143 -0.342857 -0.328571 -0.314286 -0.3 -0.285714 -0.271429 -0.257143 -0.242857 -0.228571 -0.214286 -0.2 -0.185714 -0.171429 -0.165068 -0.165068 -0.165068 -0.165068 -0.165068 -0.165068